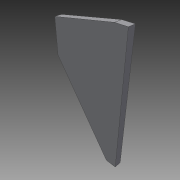
# Autodesk Inventor part: front_panel_brace_middle
Saved by Autodesk Inventor 2014 (Build 180170000, 170)
## iProperties
Created: 2014-03-23
Part Number: front_panel_brace_middle
Material: Generic
Document SubType Name: Modeling
Designer: buben
Density: 1 g/cm^3
Appearance: Default
Author: buben
Autodesk Inventor part; units mm, degrees
ref_plane "YZ Plane" through (0, 0, 0) normal (1, 0, 0) x (0, 1, 0)
ref_plane "XZ Plane" through (0, 0, 0) normal (0, 1, 0) x (-1, 0, 0)
ref_plane "XY Plane" through (0, 0, 0) normal (0, 0, 1) x (1, 0, 0)
sketch "Sketch1" plane through (0, 0, 0) normal (0, 1, 0) x (-1, 0, 0)
  line L0 (0, 0) -> (10, 0)
  line L1 (10, 0) -> (66.654, -9.9896)
  line L2 (66.654, -9.9896) -> (66.654, -41.5096)
  line L3 (66.654, -41.5096) -> (10, -122.4199)
  line L4 (10, -122.4199) -> (0, -122.4199)
  line L5 (0, -122.4199) -> (0, 0)
  dimension "d0" = 31.52
  dimension "d1" = 145
  dimension "d2" = 100
  dimension "d3" = 10
  dimension "d4" = 10
  dimension "d5" = 66.654
  constraints: 12 end point, 2 parallel, 1 horizontal, 1 perpendicular
  measures "d0" distance of L1.end L2.end
  measures "d1" angle of L3 L2
  measures "d2" angle of L1 L2
  measures "d3" distance of L0.start L0.end
  measures "d4" distance of L3.end L4.end
  measures "d5" distance between parallel lines of L5 L2
extrude "Extrusion1" add sketch "Sketch1" along normal blind 6.5
equation "\"d4\" = d3"
body "Solid1"
